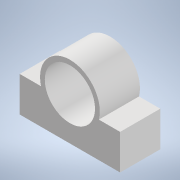
# Autodesk Inventor part: bearing housing front
Saved by Autodesk Inventor 2022.2 (Build 262287010, 287A)
## iProperties
Created: 2022-03-18
Part Number: bearing housing front
Material: Generic
Document SubType Name: Modeling
Designer: Finn Oriwohl
Density: 1 g/cm^3
Appearance: Default
Author: Finn Oriwohl
Autodesk Inventor part; units mm, degrees
ref_plane "YZ Plane" through (0, 0, 0) normal (1, 0, 0) x (0, 1, 0)
ref_plane "XZ Plane" through (0, 0, 0) normal (0, 1, 0) x (-1, 0, 0)
ref_plane "XY Plane" through (0, 0, 0) normal (0, 0, 1) x (1, 0, 0)
sketch "Sketch1" plane through (0, 0, 0) normal (0, 0, 1) x (1, 0, 0)
  line L0 (-10, 3.5) -> (10, 3.5)
  line L1 (10, 3.5) -> (10, -3.5)
  line L2 (10, -3.5) -> (-10, -3.5)
  line L3 (-10, -3.5) -> (-10, 3.5)
  line L4 (-10, 3.5) -> (10, -3.5) construction
  line L5 (10, 3.5) -> (-10, -3.5) construction
  circle A0 centre (0, 5) radius 5.9513
  circle A1 centre (0, 5) radius 5
  point P0 (0, 0)
  point P1 (5.7592, 3.5)
  point P2 (-5.7592, 3.5)
  dimension "d0" = 20
  dimension "d1" = 7
  dimension "d2" = 10
  constraints: 12 end point, 2 centre point, 2 midpoint, 2 parallel, 1 coincident, 1 horizontal, 1 perpendicular
  measures "d0" distance of L1.end L2.end
  measures "d1" distance of L0.end L1.end
  measures "d2" diameter of A1
extrude "Extrusion1" add sketch "Sketch1" along normal blind 8 contours L0 A0 L1 L2 L3 | A0 L0 A1 | L0 A1 A0
body "Solid1"
